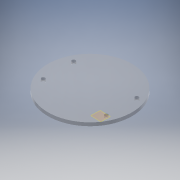
# Autodesk Inventor part: top_cover
Saved by Autodesk Inventor 2016 (Build 200138000, 138)
## iProperties
Created: 2016-09-24
Part Number: top_cover
Material: Generic
Document SubType Name: Modeling
Designer: benja
Density: 1 g/cm^3
Appearance: Polycarbonate - Clear
Author: benja
Autodesk Inventor part; units mm, degrees
ref_plane "YZ Plane" through (0, 0, 0) normal (1, 0, 0) x (0, 1, 0)
ref_plane "XZ Plane" through (0, 0, 0) normal (0, 1, 0) x (-1, 0, 0)
ref_plane "XY Plane" through (0, 0, 0) normal (0, 0, 1) x (1, 0, 0)
ref_plane "Work Plane1" through (48.8619, 11.5956, -9.64) normal (0, 1, 0) x (0.9993444, 0, 0.0362049)
sketch "Sketch1" plane through (49.7536, -1.7578, 0) normal (0, 0, 1) x (-0.9993444, 0.0362049, 0)
  arc A0 (3.3176, 0.3625) -> (1.2465, 2.2888) centre (1.3189, 0.2901) ccw projected
  line L0 (1.2465, 2.2888) -> (-3.8002, 2.106) projected
  arc A1 (-3.8002, 2.106) -> (-5.7265, 0.0349) centre (-3.7278, 0.1073) ccw projected
  line L1 (-5.7265, 0.0349) -> (-5.5816, -3.9625) projected
  arc A2 (-5.5816, -3.9625) -> (-3.5105, -5.8888) centre (-3.583, -3.8901) ccw projected
  line L2 (-3.5105, -5.8888) -> (1.5361, -5.7059) projected
  arc A3 (1.5361, -5.7059) -> (3.4624, -3.6348) centre (1.4637, -3.7073) ccw projected
  line L3 (3.4624, -3.6348) -> (3.3176, 0.3625) projected
  circle A4 centre (-1.132, -1.8) radius 1.75 projected
  arc A5 (45.1177, 3.8782) -> (43.1914, 1.8071) centre (45.1901, 1.8795) ccw projected
  line L4 (43.1914, 1.8071) -> (43.3363, -2.1903) projected
  arc A6 (43.3363, -2.1903) -> (45.4074, -4.1166) centre (45.335, -2.1179) ccw projected
  line L5 (45.4074, -4.1166) -> (50.4541, -3.9337) projected
  arc A7 (50.4541, -3.9337) -> (52.3803, -1.8626) centre (50.3816, -1.935) ccw projected
  line L6 (52.3803, -1.8626) -> (52.2355, 2.1348) projected
  arc A8 (52.2355, 2.1348) -> (50.1644, 4.061) centre (50.2368, 2.0623) ccw projected
  line L7 (50.1644, 4.061) -> (45.1177, 3.8782) projected
  circle A9 centre (47.7859, -0.0278) radius 1.75 projected
  arc A10 (44.352, -30.2274) -> (46.4231, -32.1537) centre (46.3507, -30.155) ccw projected
  line L8 (46.4231, -32.1537) -> (51.4698, -31.9708) projected
  arc A11 (51.4698, -31.9708) -> (53.3961, -29.8997) centre (51.3974, -29.9721) ccw projected
  line L9 (53.3961, -29.8997) -> (53.2513, -25.9024) projected
  arc A12 (53.2513, -25.9024) -> (51.1802, -23.9761) centre (51.2526, -25.9748) ccw projected
  line L10 (51.1802, -23.9761) -> (46.1335, -24.1589) projected
  arc A13 (46.1335, -24.1589) -> (44.2072, -26.23) centre (46.2059, -26.1576) ccw projected
  line L11 (44.2072, -26.23) -> (44.352, -30.2274) projected
  circle A14 centre (48.8016, -28.0649) radius 1.75 projected
  arc A15 (2.5519, -33.7431) -> (4.4782, -31.672) centre (2.4795, -31.7444) ccw projected
  line L12 (4.4782, -31.672) -> (4.3334, -27.6746) projected
  arc A16 (4.3334, -27.6746) -> (2.2623, -25.7483) centre (2.3347, -27.747) ccw projected
  line L13 (2.2623, -25.7483) -> (-2.7844, -25.9311) projected
  arc A17 (-2.7844, -25.9311) -> (-4.7107, -28.0022) centre (-2.712, -27.9298) ccw projected
  line L14 (-4.7107, -28.0022) -> (-4.5659, -31.9996) projected
  arc A18 (-4.5659, -31.9996) -> (-2.4948, -33.9259) centre (-2.5672, -31.9272) ccw projected
  line L15 (-2.4948, -33.9259) -> (2.5519, -33.7431) projected
  circle A19 centre (-0.1163, -29.8371) radius 1.75 projected
  circle A20 centre (39.7859, -28.0278) radius 1.75 projected
  circle A21 centre (3.1641, -28.0278) radius 1.75 projected
  circle A22 centre (11.1641, -0.0278) radius 1.75 projected
  circle A23 centre (47.7859, -0.0278) radius 1.75 projected
  line L16 (55.7859, 3.4722) -> (55.7859, -31.5278) projected
  arc A24 (55.7859, 3.4722) -> (-4.8359, 3.4722) centre (25.475, -14.0278) ccw projected
  line L17 (-4.8359, -31.5278) -> (-4.8359, 3.4722) projected
  arc A25 (-4.8359, -31.5278) -> (55.7859, -31.5278) centre (25.475, -14.0278) ccw projected
  circle A26 centre (25.475, -14.0278) radius 40
  point P0 (49.7846, 0.0447)
  dimension "d0" = 80
  constraints: 5 coincident, 1 centre point
  measures "d0" diameter of A26
extrude "Extrusion1" add sketch "Sketch1" along normal blind 3.175 contours L3 A3 L2 A2 L17 A1 L0 A0 | A0 L0 A1 L17 A24 L16 A25 A18 L15 A15 L12 A21 A16 L13 A17 L14 A2 L2 A3 L3 | L17 A2 L1 A1 | A25 A18 L14 | L14 A17 L13 A16 A21 L12 A15 L15 A18 A25 | A21 L12 A16 | A16 L12 A21 | A4 | L7 A8 L6 A7 L5 A6 L4 A5 | A9 | L11 A13 L10 A12 L9 A11 L8 A10 | A14 | A19 | A20 | A22 | A26
sketch "Sketch2" plane through (24.8031, 13.1831, 3.175) normal (0, 0, 1) x (1, 0, 0)
  circle A0 centre (-30, 14.5) radius 1.75 projected
  circle A1 centre (-30, -14.5) radius 1.75 projected
  circle A2 centre (30, -14.5) radius 1.75 projected
  circle A3 centre (30, 14.5) radius 1.75 projected
  point P0 (-24.8031, -13.1831)
  constraints: 4 coincident
hole "Hole1" at (54.8031, 27.6831, 3.175) at (54.8031, -1.3169, 3.175) at (-5.1969, -1.3169, 3.175) at (-5.1969, 27.6831, 3.175) direction (0, 0, -1) diameter 3.5 end through all
body "Solid1"
